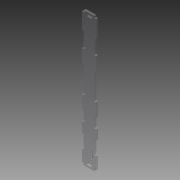
# Autodesk Inventor part: Right_wall
Saved by Autodesk Inventor 2015 (Build 190159000, 159)
## iProperties
Created: 2015-06-19
Part Number: Right_wall
Material: Generic
Document SubType Name: Modeling
Designer: Openlab
Density: 1 g/cm^3
Appearance: Polycarbonate - Clear
Author: Openlab
Autodesk Inventor part; units mm, degrees
ref_plane "YZ Plane" through (0, 0, 0) normal (1, 0, 0) x (0, 1, 0)
ref_plane "XZ Plane" through (0, 0, 0) normal (0, 1, 0) x (-1, 0, 0)
ref_plane "XY Plane" through (0, 0, 0) normal (0, 0, 1) x (1, 0, 0)
sketch "Sketch1" plane through (0, 0, 0) normal (0, 1, 0) x (-1, 0, 0)
  line L0 (21, -25) -> (18.25, -25)
  line L1 (21, -48) -> (18.25, -48)
  line L2 (21, -143) -> (18.25, -143)
  line L3 (21, -68) -> (18.25, -68)
  line L4 (21, -128) -> (18.25, -128)
  line L5 (21, -108) -> (18.25, -108)
  line L6 (2.75, -68) -> (0, -68)
  line L7 (2.75, -108) -> (0, -108)
  line L8 (2.75, -128) -> (0, -128)
  line L9 (2.75, -143) -> (0, -143)
  line L10 (2.75, -48) -> (0, -48)
  line L11 (2.75, -25) -> (0, -25)
  line L12 (21, -158) -> (21, -143)
  line L13 (21, -128) -> (21, -108)
  line L14 (21, -68) -> (21, -48)
  line L15 (21, -25) -> (21, 0)
  line L16 (0, -158) -> (0, -143)
  line L17 (0, -128) -> (0, -108)
  line L18 (0, -68) -> (0, -48)
  line L19 (0, -25) -> (0, 0)
  line L20 (18.25, -143) -> (18.25, -128)
  line L21 (18.25, -108) -> (18.25, -68)
  line L22 (18.25, -48) -> (18.25, -25)
  line L23 (2.75, -143) -> (2.75, -128)
  line L24 (2.75, -108) -> (2.75, -68)
  line L25 (2.75, -48) -> (2.75, -25)
  line L26 (21, -68) -> (21, -48) construction
  line L27 (10.5, -68) -> (10.5, -97) construction
  line L28 (18.25, -158) -> (18.25, -178)
  line L29 (18.25, -178) -> (21, -178)
  line L30 (21, -178) -> (21, -196)
  line L31 (0, -196) -> (0, -178)
  line L32 (0, -178) -> (2.75, -178)
  line L33 (2.75, -158) -> (2.75, -178)
  line L34 (21, -158) -> (18.25, -158)
  line L35 (2.75, -158) -> (0, -158)
  line L36 (7.55, -176) -> (5.75, -176)
  line L37 (5.75, -176) -> (5.75, -186)
  line L38 (5.75, -186) -> (7.55, -186)
  line L39 (7.55, -186) -> (7.55, -176)
  line L40 (18.25, 0) -> (18.25, 2.75)
  line L41 (18.25, 2.75) -> (2.75, 2.75)
  line L42 (2.75, 2.75) -> (2.75, 0)
  line L43 (21, 0) -> (18.25, 0)
  line L44 (2.75, 0) -> (0, 0)
  line L45 (18.25, -196) -> (18.25, -198.75)
  line L46 (18.25, -198.75) -> (2.75, -198.75)
  line L47 (2.75, -198.75) -> (2.75, -196)
  line L48 (21, -196) -> (18.25, -196)
  line L49 (2.75, -196) -> (0, -196)
  line L50 (14, 0) -> (7, 0)
  line L51 (7, 0) -> (7, -3)
  line L52 (7, -3) -> (14, -3)
  line L53 (14, -3) -> (14, 0)
  line L54 (14, -193) -> (7, -193)
  line L55 (7, -193) -> (7, -196)
  line L56 (7, -196) -> (14, -196)
  line L57 (14, -196) -> (14, -193)
  dimension "d7" = 23
  dimension "d8" = 20
  dimension "d9" = 40
  dimension "d10" = 20
  dimension "d11" = 15
  dimension "d28" = 15.5
  dimension "d31" = 2.75
  dimension "d44" = 18
  dimension "d45" = 20
  dimension "d47" = 15
  dimension "d49" = 1.8
  dimension "d51" = 10
  dimension "d53" = 3
  dimension "d55" = 25
  dimension "d56" = 10
  dimension "d57" = 7
  dimension "d58" = 3
  constraints: 117 end point, 34 collinear, 20 perpendicular, 8 parallel, 6 vertical, 5 equal length, 3 horizontal, 2 point on line, 5 other
  measures "d7" distance between parallel lines of L1 L0
  measures "d8" distance between parallel lines of L3 L1
  measures "d9" distance between parallel lines of L5 L3
  measures "d10" distance between parallel lines of L4 L5
  measures "d11" distance between parallel lines of L2 L4
  measures "d28" distance between parallel lines of L23 L20
  measures "d31" distance between parallel lines of L22 L15
  measures "d44" distance of L29.end L30.end
  measures "d45" distance of L28.start L28.end
  measures "d47" distance of L12.start L2.start
  measures "d49" distance of L36.start L36.end
  measures "d51" distance of L38.end L36.start
  measures "d53" distance between parallel lines of L33 L37
  measures "d55" distance of L0.start L15.end
  measures "d56" distance between parallel lines of L49 L38
  measures "d57" distance of L51.end L52.end
  measures "d58" distance of L50.end L51.end
extrude "Extrusion3" add sketch "Sketch1" along normal blind 3
body "Solid3"
